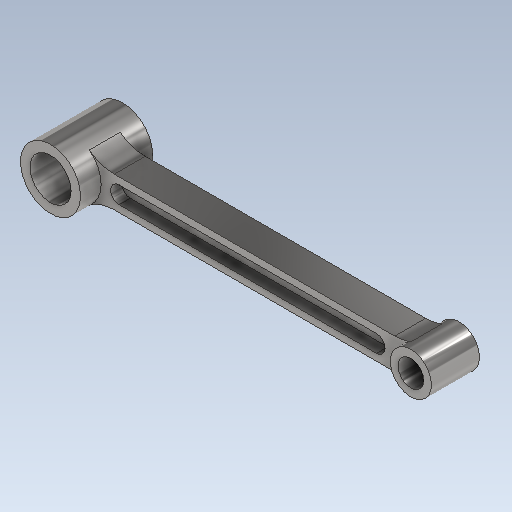
# Autodesk Inventor part: 18
Saved by Autodesk Inventor 2021 (Build 250183000, 183)
## iProperties
Category: 41
Created: 2021-07-17
Part Number: 18
Material: Aço
Document SubType Name: Modeling
Designer: Giovanni
Density: 7.85 g/cm^3
Appearance: Aço - Polido
User Status: 1:2
Description: 18
Author: Giovanni
Keywords: 3
Revision Number: 18
Autodesk Inventor part; units mm, degrees
ref_plane "YZ Plane" through (0, 0, 0) normal (1, 0, 0) x (0, 1, 0)
ref_plane "XZ Plane" through (0, 0, 0) normal (0, 1, 0) x (-1, 0, 0)
ref_plane "XY Plane" through (0, 0, 0) normal (0, 0, 1) x (1, 0, 0)
sketch "Esboço1" plane through (0, 0, 0) normal (0, 0, 1) x (1, 0, 0)
  circle A0 centre (0, 0) radius 12
  circle A1 centre (0, 0) radius 17.5
  dimension "d1" = 24
  dimension "d0" = 35
  constraints: 2 centre point, 2 coincident
  measures "d1" diameter of A0
  measures "d0" diameter of A1
extrude "Extrusão1" add sketch "Esboço1" along normal mid plane 42
sketch "Esboço2" plane through (0, 0, 0) normal (0, 0, 1) x (1, 0, 0)
  circle A0 centre (203, 0) radius 12
  circle A1 centre (203, 0) radius 7.5
  point P0 (0, 0)
  dimension "d5" = 24
  dimension "d6" = 15
  dimension "d9" = 203
  constraints: 2 centre point, 1 coincident
  measures "d5" diameter of A0
  measures "d6" diameter of A1
  measures "d9" distance of point (0, 0) A0.centre
extrude "Extrusão2" add sketch "Esboço2" along normal mid plane 28
sketch "Esboço4" plane through (0, 0, 0) normal (0, 0, 1) x (1, 0, 0)
  line L0 (7.9373, 9) -> (195.0627, 9)
  circle A0 centre (0, 0) radius 17.5 projected
  circle A1 centre (0, 0) radius 12 projected
  circle A2 centre (203, 0) radius 12 projected
  circle A3 centre (203, 0) radius 7.5 projected
  line L1 (15.0083, -9) -> (195.0627, -9)
  point P0 (15.0083, 9)
  dimension "d11" = 9
  constraints: 4 end point, 2 horizontal, 2 point on circle, 4 other
  measures "d11" distance from line of point (0, 0) L0
extrude "Extrusão3" add sketch "Esboço4" along normal mid plane 18 contours L0 A2 L1 A0
sketch "Esboço5" plane through (0, 0, 9) normal (0, 0, 1) x (1, 0, 0)
  arc A0 (28, 5) -> (28, -5) centre (28, 0) ccw
  arc A1 (178, -5) -> (178, 5) centre (178, 0) ccw
  line L0 (28, -5) -> (178, -5)
  line L1 (28, 5) -> (178, 5)
  point P0 (0, 0)
  dimension "d14" = 28
  dimension "d15" = 150
  dimension "d16" = 10
  dimension "d17" = 5
  constraints: 4 end point, 4 point on circle, 4 tangent, 2 centre point, 1 equal radius
  measures "d14" distance of point (0, 0) A0.centre
  measures "d15" distance of A1.centre A0.centre
  measures "d16" distance between parallel lines of L0 L1
  measures "d17" radius of A0
extrude "Extrusão4" cut sketch "Esboço5" against normal blind 6.5
mirror "Espelhamento1" about plane through (0, 0, 0) normal (0, 0, 1) of "Extrusão4"
fillet "Arredondamento1" radius 24 4 edges at (15.0083, 9, 0) (195.0627, 9, 0) (195.0627, -9, 0) (15.0083, -9, 0)
